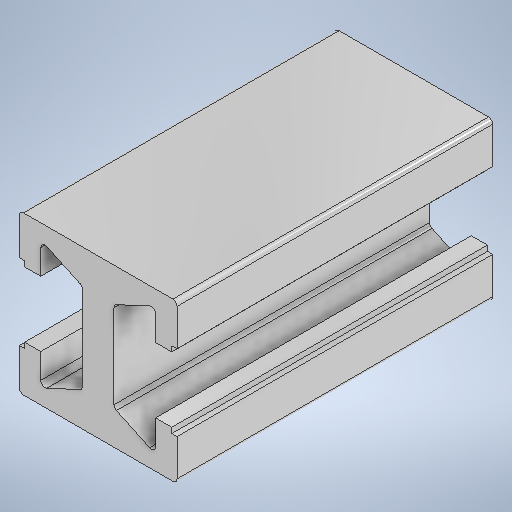
# Autodesk Inventor part: Perfil_15x15_001
Saved by Autodesk Inventor 2025.2 (Build 292293000, 293)
## iProperties
Created: 2025-03-22
Part Number: Perfil_15x15_001
Material: Alumínio 6061-AHC
Document SubType Name: Modeling
Designer: Carlos Dias
Density: 2.7 g/cm^3
Appearance: Alumínio - Polido
Author: Carlos Dias
## iProperties of the stored document Perfil_15x15_001_3DPrint.ipt
Created: 2025-03-22
Part Number: Perfil_15x15_001_3DPrint
Material: Genérico
Document SubType Name: Modeling
Designer: Carlos Dias
Density: 1 g/cm^3
Appearance: Padrão
Author: Carlos Dias
Autodesk Inventor part; units mm, degrees
ref_plane "YZ Plane" through (0, 0, 0) normal (1, 0, 0) x (0, 1, 0)
ref_plane "XZ Plane" through (0, 0, 0) normal (0, 1, 0) x (-1, 0, 0)
ref_plane "XY Plane" through (0, 0, 0) normal (0, 0, 1) x (1, 0, 0)
sketch "Esboço1" plane through (0, 0, 0) normal (0, 0, 1) x (1, 0, 0)
  line L0 (-75, 75) -> (75, 75) construction
  line L1 (0, 0) -> (0, 75) construction
  line L2 (-15, 0) -> (15, 0) construction
  line L3 (-74.6189, 31) -> (-54.6189, 31) construction
  line L4 (-74.6189, 31) -> (-74.6189, 0) construction
  line L5 (-75, 36.1611) -> (-70, 36.1611)
  line L6 (-70, 36.1611) -> (-70, 31)
  line L7 (-70, 31) -> (-54.6189, 31)
  line L8 (-75, 71) -> (-75, 36.1611)
  line L9 (-54.6189, 54.7213) -> (-54.6189, 31)
  line L10 (-15, 39.9771) -> (-15, 19.9886) construction
  line L11 (-48.9284, 58.3465) -> (-17.3095, 43.6024)
  line L12 (-54.6189, 61) -> (-19.7313, 61) construction
  line L13 (-74.6189, 0) -> (-15, 0) construction
  line L14 (-15, 42.5254) -> (-15, 0)
  line L15 (-15, 0) -> (0, 0) construction
  line L16 (0, 0) -> (0, 75)
  line L17 (71, 75) -> (-71, 75)
  line L18 (74.6189, 31) -> (54.6189, 31) construction
  line L19 (74.6189, 31) -> (74.6189, 0) construction
  line L20 (75, 36.1611) -> (70, 36.1611)
  line L21 (70, 36.1611) -> (70, 31)
  line L22 (70, 31) -> (54.6189, 31)
  line L23 (75, 71) -> (75, 36.1611)
  line L24 (54.6189, 54.7213) -> (54.6189, 31)
  line L25 (15, 75) -> (15, 19.9886) construction
  line L26 (48.9284, 58.3465) -> (17.3095, 43.6024)
  line L27 (54.6189, 61) -> (19.7313, 61) construction
  line L28 (74.6189, 0) -> (15, 0) construction
  line L29 (15, 39.9771) -> (15, 0)
  line L30 (15, 0) -> (0, 0) construction
  line L31 (-71, -75) -> (71, -75)
  line L32 (0, 0) -> (0, -75) construction
  line L33 (-74.6189, -31) -> (-54.6189, -31) construction
  line L34 (-74.6189, -31) -> (-74.6189, 0) construction
  line L35 (-75, -36.1611) -> (-70, -36.1611)
  line L36 (-70, -36.1611) -> (-70, -31)
  line L37 (-70, -31) -> (-54.6189, -31)
  line L38 (-75, -71) -> (-75, -36.1611)
  line L39 (-54.6189, -54.7213) -> (-54.6189, -31)
  line L40 (-15, -75) -> (-15, -19.9886) construction
  line L41 (-48.9284, -58.3465) -> (-17.3095, -43.6024)
  line L42 (-54.6189, -61) -> (-19.7313, -61) construction
  line L43 (-75, -71) -> (-75, 0) construction
  line L44 (-15, -39.9771) -> (-15, 0)
  line L45 (0, 0) -> (0, -75)
  line L46 (74.6189, -31) -> (74.6189, 0) construction
  line L47 (70, -31) -> (54.6189, -31)
  line L48 (70, -36.1611) -> (70, -31)
  line L49 (74.6189, -31) -> (54.6189, -31) construction
  line L50 (75, -36.1611) -> (70, -36.1611)
  line L51 (75, -75) -> (75, 0) construction
  line L52 (75, -71) -> (75, -36.1611)
  line L53 (54.6189, -54.7213) -> (54.6189, -31)
  line L54 (48.9284, -58.3465) -> (17.3095, -43.6024)
  line L55 (54.6189, -61) -> (19.7313, -61) construction
  line L56 (15, -42.5254) -> (15, 0)
  line L57 (15, -39.9771) -> (15, 0) construction
  line L58 (75, -75) -> (-75, -75) construction
  arc A0 (-48.9284, 58.3465) -> (-54.6189, 54.7213) centre (-50.6189, 54.7213) ccw
  arc A1 (-15, 39.9771) -> (-17.3095, 43.6024) centre (-19, 39.9771) ccw
  arc A2 (-17.3095, -43.6024) -> (-15, -39.9771) centre (-19, -39.9771) ccw
  arc A3 (-54.6189, -54.7213) -> (-48.9284, -58.3465) centre (-50.6189, -54.7213) ccw
  arc A4 (48.9284, -58.3465) -> (54.6189, -54.7213) centre (50.6189, -54.7213) ccw
  arc A5 (15, -39.9771) -> (17.3095, -43.6024) centre (19, -39.9771) ccw
  arc A6 (54.6189, 54.7213) -> (48.9284, 58.3465) centre (50.6189, 54.7213) ccw
  arc A7 (17.3095, 43.6024) -> (15, 39.9771) centre (19, 39.9771) ccw
  arc A8 (-71, 75) -> (-75, 71) centre (-71, 71) ccw
  arc A9 (75, 71) -> (71, 75) centre (71, 71) ccw
  arc A10 (71, -75) -> (75, -71) centre (71, -71) ccw
  arc A11 (-75, -71) -> (-71, -75) centre (-71, -71) ccw
  arc A12 (-75, -71) -> (-71, -75) centre (-71, -71) ccw
  point P0 (-15, 75)
  point P1 (15, 42.5254)
  point P2 (-15, -42.5254)
  point P3 (15, -75)
  point P4 (15, -39.9771)
  dimension "d0" = 150
  dimension "d4" = 20
  dimension "d6" = 31
  dimension "d7" = 5
  dimension "d8" = 44
  dimension "d9" = 38.8389
  dimension "d11" = 30
  dimension "d13" = 20.3811
  dimension "d14" = 25
  dimension "d20" = 4
  dimension "d21" = 4
  dimension "d22" = 4
  dimension "d23" = 4
  dimension "d25" = 15
  constraints: 118 end point, 40 point on line, 37 symmetric about line, 26 point on circle, 26 tangent, 13 centre point, 9 equal radius, 7 horizontal alignment, 6 horizontal, 6 vertical, 4 midpoint, 4 vertical alignment, 3 perpendicular, 2 coincident, 2 equal length
  measures "d0" distance of L0.start L0.end
  measures "d4" distance of L3.start L3.end
  measures "d6" distance of L3.start L4.end
  measures "d7" distance of L5.start L5.end
  measures "d8" distance between parallel lines of L0 L3
  measures "d9" distance from line of L0 L5.end
  measures "d11" distance of L12.start L3.end
  measures "d13" distance between parallel lines of L8 L9
  measures "d14" angle of L11 L12
  measures "d20" radius of A0
  measures "d21" radius of A8
  measures "d22" radius of A9
  measures "d23" radius of A12
  measures "d25" distance between parallel lines of L1 L14
extrude "Extrusão2" add sketch "Esboço1" against normal blind 300
